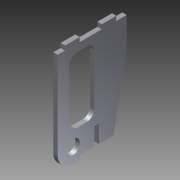
# Autodesk Inventor part: OpenROV 2_2 Handel
Saved by Autodesk Inventor 2011 (Build 150239000, 239)
## iProperties
Created: 2011-12-01
Part Number: OpenROV 2_2 Handel
Document SubType Name: Modeling
Designer: user
Density: 1 g/cm^3
Author: user
Autodesk Inventor part; units mm, degrees
ref_plane "YZ Plane" through (0, 0, 0) normal (1, 0, 0) x (0, 1, 0)
ref_plane "XZ Plane" through (0, 0, 0) normal (0, 1, 0) x (-1, 0, 0)
ref_plane "XY Plane" through (0, 0, 0) normal (0, 0, 1) x (1, 0, 0)
sketch "Sketch1" plane through (0, 0, 0) normal (0, 0, 1) x (1, 0, 0)
  line L0 (8.95, -66.5) -> (18.95, -66.5)
  line L1 (18.95, -66.5) -> (18.95, -54.5)
  line L2 (18.95, -54.5) -> (21.95, -54.5)
  line L3 (21.95, -54.5) -> (21.95, -66.5)
  line L4 (31.95, -69.5) -> (36.95, -69.5)
  line L5 (46.95, -59.5) -> (46.95, 0)
  arc A0 (36.95, -69.5) -> (46.95, -59.5) centre (36.95, -59.5) ccw
  line L6 (26.95, -5) -> (33.95, -5)
  line L7 (38.95, -10) -> (38.95, -44.5)
  line L8 (33.95, -49.5) -> (26.95, -49.5)
  line L9 (21.95, -44.5) -> (21.95, -10)
  circle A1 centre (36.95, -59.5) radius 5
  arc A2 (21.95, -44.5) -> (26.95, -49.5) centre (26.95, -44.5) ccw
  arc A3 (33.95, -49.5) -> (38.95, -44.5) centre (33.95, -44.5) ccw
  arc A4 (38.95, -10) -> (33.95, -5) centre (33.95, -10) ccw
  arc A5 (26.95, -5) -> (21.95, -10) centre (26.95, -10) ccw
  line L10 (16.95, 0) -> (16.95, 3)
  line L11 (16.95, 3) -> (6.95, 3)
  line L12 (6.95, 3) -> (6.95, 0)
  line L13 (31.95, 0) -> (31.95, 3)
  line L14 (31.95, 3) -> (41.95, 3)
  line L15 (41.95, 3) -> (41.95, 0)
  line L16 (46.95, 0) -> (41.95, 0)
  line L17 (31.95, 0) -> (16.95, 0)
  line L18 (6.95, 0) -> (0, 0)
  line L19 (0, 0) -> (0, -21.8009)
  line L20 (21.95, -66.5) -> (31.95, -66.5)
  line L21 (31.95, -66.5) -> (31.95, -69.5)
  line L22 (8.95, -66.5) -> (0.0393, -22.1952)
  arc A6 (0, -21.8009) -> (0.0393, -22.1952) centre (2, -21.8009) ccw
  point P0 (46.95, -69.5)
  point P1 (0, -22)
  dimension "d7" = 10
  dimension "d8" = 8
  dimension "d11" = 20
  dimension "d12" = 10
  dimension "d14" = 5
  dimension "d17" = 10
  dimension "d18" = 3
  dimension "d20" = 10
  dimension "d21" = 3
  dimension "d22" = 5
  dimension "d23" = 15
  dimension "d24" = 3
  dimension "d25" = 3
  dimension "d26" = 69.5
  dimension "d27" = 5
  dimension "d31" = 3
  dimension "d36" = 18.95
  dimension "d40" = 3
  dimension "d41" = 10
  dimension "d42" = 3
  dimension "d43" = 15
  dimension "d44" = 21.95
  dimension "d46" = 6.95
  dimension "d47" = 22
  dimension "d48" = 10
  dimension "d49" = 2
  dimension "d51" = 12
  dimension "d52" = 66.5
  constraints: 46 end point, 12 point on circle, 12 tangent, 9 parallel, 7 centre point, 4 point on line, 3 equal radius, 3 perpendicular, 1 coincident, 1 horizontal
  measures "d7" radius of A0
  measures "d8" distance between parallel lines of L5 L7
  measures "d11" distance between parallel lines of L4 L8
  measures "d12" diameter of A1
  measures "d14" radius of A2
  measures "d17" distance of L10.end L11.end
  measures "d18" distance of L11.end L12.end
  measures "d20" distance of L13.end L14.end
  measures "d21" distance of L14.end L15.end
  measures "d22" distance between parallel lines of L5 L15
  measures "d23" distance of L13.start L10.start
  measures "d24" distance of L10.start L10.end
  measures "d25" distance of L13.start L13.end
  measures "d26" distance between parallel lines of L17 L4
  measures "d27" distance between parallel lines of L17 L6
  measures "d31" distance between parallel lines of L0 L4
  measures "d36" distance between parallel lines of L19 L1
  measures "d40" distance of L20.end L4.start
  measures "d41" distance of L3.end L20.end
  measures "d42" distance between parallel lines of L1 L3
  measures "d43" distance between parallel lines of L21 L5
  measures "d44" distance between parallel lines of L19 L9
  measures "d46" distance between parallel lines of L19 L12
  measures "d47" distance of L18.end point (0, -22)
  measures "d48" distance of L0.start L0.end
  measures "d49" radius of A6
  measures "d51" distance between parallel lines of L0 L2
  measures "d52" distance between parallel lines of L0 L18
extrude "Extrusion1" add sketch "Sketch1" along normal blind 3
body "Solid1"
